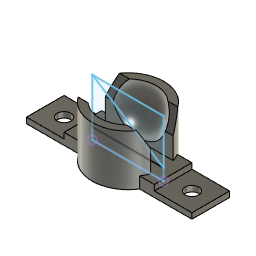
robot (Autodesk Fusion 360 archive; units mm, degrees)
design "Back Caster"
Autodesk Fusion 360 part; units mm, degrees
sketch "Sketch1" plane through (0, 0, 0) normal (0, 0, 1) x (1, 0, 0)
  circle A0 centre (0, 0) radius 9.5
  line L0 (12, 5) -> (-12, 5)
  line L1 (-12, 5) -> (-12, -5)
  line L2 (-12, -5) -> (12, -5)
  line L3 (12, -5) -> (12, 5)
  line L4 (-12, -5) -> (-22, -5)
  line L5 (-22, -5) -> (-22, 5)
  line L6 (-22, 5) -> (-12, 5)
  line L7 (-12, 5) -> (-12, -5)
  line L8 (12, -5) -> (22, -5)
  line L9 (22, -5) -> (22, 5)
  line L10 (22, 5) -> (12, 5)
  line L11 (12, 5) -> (12, -5)
  circle A1 centre (17, 0) radius 1.825
  circle A2 centre (-17, 0) radius 1.825
  dimension "d1" = 19
  dimension "d2" = 5
  dimension "d3" = 5
  dimension "d4" = 12
  dimension "d19" = 24
  dimension "d20" = 3.65
  dimension "d21" = 3.65
  constraint coincident A0.centre origin
  constraint horizontal L0
  constraint vertical L1
  constraint horizontal L2
  constraint vertical L3
  constraint horizontal L4
  constraint vertical L5
  constraint horizontal L6
  constraint vertical L7
  constraint horizontal L8
  constraint vertical L9
  constraint horizontal L10
  constraint vertical L11
  measures "d1" diameter of A0
  measures "d2" distance of A0.centre L0
  measures "d3" distance of A0.centre L2
  measures "d4" distance of A0.centre L3
  measures "d19" distance of L1 L3
  measures "d20" diameter of A1
  measures "d21" diameter of A2
extrude "Extrude1" add sketch "Sketch1" along normal blind 3 contours A0 L0 L2 L3 L11 | A0 L0 L1 L2 L7 makes body 1 at (-9.0078, 3.0183, 2) makes body 2 at (8.3, 4.6217, 2)
extrude "Extrude2" add sketch "Sketch1" along normal blind 13.5 contours A0 L0 L2 | A0 L0 | A0 L2 bodies 1 2
sketch "Sketch2" plane through (0, 0, 0) normal (0, 1, 0) x (1, 0, 0)
  line L0 (-9.5, -15) -> (9.5, -15)
  line L1 (9.5, -15) -> (9.5, 0)
  line L2 (9.5, 0) -> (-9.5, 0)
  line L3 (-9.5, 0) -> (-9.5, -15)
  line L4 (9.5, 0) -> (-9.5, 0)
  line L5 (-9.5, 0) -> (-9.5, -3)
  line L6 (-9.5, -3) -> (9.5, -3)
  line L7 (9.5, -3) -> (9.5, 0)
  line L8 (-9.5, -15) -> (9.5, -3)
  line L9 (-9.5, 0) -> (9.5, 0)
  dimension "d10" = 3
  constraint horizontal L0
  constraint vertical L1
  constraint horizontal L2
  constraint vertical L3
  constraint horizontal L4
  constraint vertical L5
  constraint horizontal L6
  constraint vertical L7
  constraint coincident L3 L5.end
  measures "d10" distance of L6 L9
sphere "SpherePrimitive2" cut diameter 15.8 placed x (1, 0, 0) y (0, 0, -1) z (0, 1, 0) at (0, 0, 11) bodies 1
sketch "Sketch7" plane through (0, 0, 0) normal (1, 0, 0) x (0, 1, 0)
  line L0 (0, 3) -> (-3, 3)
  line L1 (-3, 3) -> (-3, 13.5)
  line L2 (-3, 13.5) -> (0, 13.5)
  line L3 (0, 13.5) -> (0, 3)
  line L4 (-5, 0) -> (-5, 3)
  line L5 (0, 15) -> (0, 0)
  line L6 (0, 3) -> (3, 3)
  line L7 (3, 3) -> (3, 13.5)
  line L8 (0, 13.5) -> (0, 3)
  line L9 (3, 13.5) -> (0, 13.5)
  line L10 (0, 13.5) -> (-5.5, 13.5)
  line L11 (-5.5, 13.5) -> (0, 3)
  line L12 (5.5, 13.5) -> (0, 3)
  line L13 (0, 13.5) -> (5.5, 13.5)
  dimension "d12" = 3
  dimension "d13" = 2
  dimension "d14" = 10.5
  constraint horizontal L0
  constraint vertical L1
  constraint horizontal L2
  constraint vertical L3
  constraint symmetric L0.start L5 L3.end
  constraint symmetric L0.end L5 L6.end
  constraint symmetric L1.end L5 L7.end
  constraint symmetric L2.end L5 L3.start
  constraint perpendicular L1 L10
  constraint symmetric L5 L0.start L3.end
  constraint symmetric L5 L10.end L12.start
  measures "d12" distance of L0.start L0.end
  measures "d13" distance of L1 L4
  measures "d14" distance of L0 L2
extrude "Extrude3" cut sketch "Sketch7" along normal blind 17 bodies 1
extrude "Extrude4" cut sketch "Sketch7" against normal blind 11 bodies 1
extrude "Extrude5" add sketch "Sketch1" along normal blind 1.5 contours L3 L8 L9 L10 L11 | L1 L4 L5 L6 L7 bodies 1
equation "d1 = 15 mm + 4 mm"

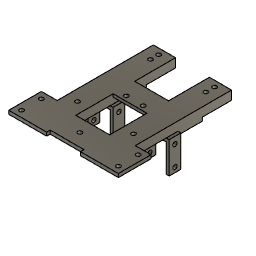
design "Dual Motor Mount"
Autodesk Fusion 360 part; units mm, degrees
sketch "Base" plane through (0, 0, 0) normal (0, 0, 1) x (1, 0, 0)
  line L0 (0, 0) -> (19, 0)
  line L1 (19, 0) -> (19, 31)
  line L2 (19, 31) -> (0, 31)
  line L3 (0, 31) -> (0, 0)
  line L4 (19, 0) -> (21.5, 0)
  line L5 (21.5, 0) -> (21.5, 10)
  line L6 (21.5, 10) -> (19, 10)
  line L7 (19, 10) -> (19, 0)
  line L8 (0, 0) -> (-2.5, 0)
  line L9 (-2.5, 0) -> (-2.5, 10)
  line L10 (-2.5, 10) -> (0, 10)
  line L11 (0, 10) -> (0, 0)
  line L12 (0, 2.5) -> (19, 2.5)
  line L13 (0, 12.6795) -> (0, 2.5)
  line L14 (0, 21) -> (19, 21)
  dimension "d1" = 19
  dimension "d2" = 31
  dimension "d3" = 2.5
  dimension "d4" = 10
  dimension "d5" = 2.5
  dimension "d6" = 10
  dimension "d8" = 2.5
  dimension "d9" = 10
  constraint horizontal L0
  constraint vertical L1
  constraint horizontal L2
  constraint vertical L3
  constraint coincident L0.start L3.end
  constraint horizontal L4
  constraint vertical L5
  constraint horizontal L6
  constraint vertical L7
  constraint horizontal L8
  constraint vertical L9
  constraint horizontal L10
  constraint vertical L11
  constraint coincident L11 L12.start
  constraint coincident L1 L12.end
  constraint vertical L13
  constraint coincident L3 L14.start
  constraint coincident L1 L14.end
  constraint perpendicular L1 L14
  measures "d1" distance of L0.start L0.end
  measures "d2" distance of L0.start L2.end
  measures "d3" distance of L0.end L4.end
  measures "d4" distance of L0.end L6.end
  measures "d5" distance of L0.start L8.end
  measures "d6" distance of L0.start L10.end
  measures "d8" distance of L0 L12
  measures "d9" distance of L2 L14
extrude "Extrude1" add sketch "Base" along normal blind 3 makes body 1
extrude "Extrude2" add sketch "Base" along normal blind 8 separate body contours L1 L3 L7 L11 L12 L13 L14 makes body 2
extrude "Extrude3" add sketch "Base" against normal blind 24 contours L3 L8 L9 L10 L11 L13 | L1 L4 L5 L6 L7 bodies 1 2
sketch "Sensor mount" plane through (0, 0, 8) normal (0, 0, 1) x (-1, 0, 0)
  line L0 (0, -21) -> (0, -2.5)
  line L1 (0, -2.5) -> (-19, -2.5)
  line L2 (-19, -2.5) -> (-19, -21)
  line L3 (-19, -21) -> (0, -21)
  line L4 (-19, -21) -> (-33.5, -21)
  line L5 (-33.5, -21) -> (-33.5, -2.5)
  line L6 (-33.5, -2.5) -> (-19, -2.5)
  line L7 (-19, -2.5) -> (-19, -21)
  line L8 (-33.5, -2.5) -> (-33.5, -21)
  line L9 (-19, -6.5) -> (-33.5, -6.5)
  circle A0 centre (-26.25, -6.5) radius 1.825
  dimension "d16" = 14.5
  dimension "d17" = 18.5
  dimension "d19" = 4
  dimension "d20" = 3.65
  constraint horizontal L4
  constraint vertical L5
  constraint horizontal L6
  constraint vertical L7
  constraint coincident L2.end L3.start
  constraint vertical L8
  constraint coincident L7 L9.start
  constraint coincident L8 L9.end
  constraint perpendicular L8 L9
  constraint midpoint L9 A0.centre
  measures "d16" distance of L2.end L4.end
  measures "d17" distance of L2.end L1.end
  measures "d19" distance of L6 L9
  measures "d20" diameter of A0
extrude "Extrude4" add sketch "Sensor mount" along normal blind 2.6 contours L0 L1 L2 L3 L7 | L2 L4 L5 L7 L8 L9 A0 | L2 L5 L6 L7 L8 L9 A0 bodies 1
sketch "Motor Holes" plane through (21.5, 0, 0) normal (1, 0, 0) x (0, 1, 0)
  line L0 (10, -24) -> (10, 3)
  line L1 (10, 3) -> (0, 3)
  line L2 (0, 3) -> (0, -24)
  line L3 (0, -24) -> (10, -24)
  line L4 (0, 0) -> (10, 0)
  circle A0 centre (5, -2.825) radius 1.825
  line L5 (5, -4.65) -> (5, -18)
  circle A1 centre (5, -19.825) radius 1.825
  line L6 (0, -2.825) -> (3.175, -2.825)
  line L7 (6.825, -2.825) -> (10, -2.825)
  dimension "d25" = 2.825
  dimension "d26" = 3.65
  dimension "d27" = 17
  dimension "d28" = 3.65
  constraint coincident L4.start origin
  constraint coincident L0 L4.end
  constraint perpendicular L0 L4
  constraint coincident L2 L6.start
  constraint coincident L0 L7.end
  constraint perpendicular L0 L6
  constraint perpendicular L5 L6
  constraint coincident A0 L6.end
  constraint collinear L6 L7
  constraint coincident A0.centre L6
  constraint coincident A0 L7.start
  constraint coincident A0 L5.start
  constraint coincident A1 L5.end
  measures "d25" distance of L4 L6
  measures "d26" diameter of A0
  measures "d27" distance of A0.centre A1.centre
  measures "d28" diameter of A1
extrude "Extrude6" cut sketch "Motor Holes" against normal blind 30 contours A0 | A1 bodies 1
sketch "Version" plane through (0, 0, 10.6) normal (0, 0, 1) x (-1, 0, 0)
  circle A0 centre (-26.25, -6.5) radius 1.825
  line L0 (-33.5, -21) -> (0, -21)
  line L1 (0, -21) -> (0, -2.5)
  line L2 (0, -2.5) -> (-33.5, -2.5)
  line L3 (-3, -14) -> (-16, -14) construction
  line L4 (-16, -14) -> (-16, -19) construction
  line L5 (-16, -19) -> (-3, -19) construction
  line L6 (-3, -19) -> (-3, -14) construction
  line L7 (-33.5, -2.5) -> (-33.5, -21)
  dimension "d31" = 8
mirror "Mirror1" about plane through (0, 0, 0) normal (1, 0, 0) of bodies 1 makes body 3
move_body "Move1" bodies 3 to x (1, 0, 0) y (0, 1, 0) z (0, 0, 1) at (67, 0, 0)
combine "Combine1" operation add target body 3 tool bodies 1
sketch "Sketch5" plane through (0, 2.5, 0) normal (0, -1, 0) x (1, 0, 0)
  line L0 (48, 3) -> (67, 3)
  line L1 (67, 3) -> (67, 10.6)
  line L2 (67, 10.6) -> (0, 10.6)
  line L3 (0, 10.6) -> (0, 3)
  line L4 (0, 3) -> (19, 3)
  line L5 (19, 3) -> (19, 8)
  line L6 (19, 8) -> (48, 8)
  line L7 (48, 8) -> (48, 3)
  line L8 (0, 10.6) -> (19, 10.6)
  line L9 (19, 10.6) -> (19, 3)
  line L10 (19, 3) -> (0, 3)
  line L11 (0, 3) -> (0, 10.6)
  line L12 (67, 3) -> (48, 3)
  line L13 (48, 3) -> (48, 10.6)
  line L14 (48, 10.6) -> (67, 10.6)
  line L15 (67, 10.6) -> (67, 3)
  constraint horizontal L8
  constraint vertical L9
  constraint horizontal L10
  constraint vertical L11
  constraint coincident L4.end L5.start
  constraint coincident L2.end L3.start
  constraint horizontal L12
  constraint vertical L13
  constraint horizontal L14
  constraint vertical L15
  constraint coincident L2 L13.end
  constraint coincident L0.end L1.start
extrude "Extrude8" add sketch "Sketch5" along normal blind 32 contours L0 L1 L2 L7 L12 L13 L14 L15 | L2 L3 L4 L5 L8 L9 L10 L11 bodies 3
sketch "Sketch6" plane through (0, 0, 10.6) normal (0, 0, 1) x (-1, 0, 0)
  circle A0 centre (-26.25, -6.5) radius 1.825
  circle A1 centre (-40.75, -6.5) radius 1.825
  line L0 (-67, -21) -> (0, -21)
  line L1 (0, -21) -> (0, 29.5)
  line L2 (0, 29.5) -> (-19, 29.5)
  line L3 (-19, 29.5) -> (-19, -2.5)
  line L4 (-19, -2.5) -> (-48, -2.5)
  line L5 (-48, -2.5) -> (-48, 29.5)
  line L6 (-48, 29.5) -> (-67, 29.5)
  line L7 (-67, 29.5) -> (-67, -21)
  line L8 (-67, 29.5) -> (-77.5, 29.5)
  line L9 (-77.5, 29.5) -> (-77.5, 51.5)
  line L10 (-77.5, 51.5) -> (-67, 51.5)
  line L11 (-67, 51.5) -> (-67, 29.5)
  line L12 (-77.5, 51.5) -> (10.5, 51.5)
  line L13 (10.5, 51.5) -> (10.5, 29.5)
  line L14 (10.5, 29.5) -> (-77.5, 29.5)
  line L15 (-77.5, 29.5) -> (-77.5, 51.5)
  line L16 (10.5, 29.5) -> (8, 29.5)
  line L17 (8, 29.5) -> (8, 32)
  line L18 (8, 32) -> (10.5, 32)
  line L19 (10.5, 32) -> (10.5, 29.5)
  line L20 (10.5, 51.5) -> (8, 51.5)
  line L21 (8, 51.5) -> (8, 49)
  line L22 (8, 49) -> (10.5, 49)
  line L23 (10.5, 49) -> (10.5, 51.5)
  line L24 (-77.5, 51.5) -> (-75, 51.5)
  line L25 (-75, 51.5) -> (-75, 49)
  line L26 (-75, 49) -> (-77.5, 49)
  line L27 (-77.5, 49) -> (-77.5, 51.5)
  line L28 (-77.5, 29.5) -> (-75, 29.5)
  line L29 (-75, 29.5) -> (-75, 32)
  line L30 (-75, 32) -> (-77.5, 32)
  line L31 (-77.5, 32) -> (-77.5, 29.5)
  circle A2 centre (8, 32) radius 1.8
  circle A3 centre (8, 49) radius 1.8
  circle A4 centre (-75, 49) radius 1.8
  circle A5 centre (-75, 32) radius 1.8
  line L32 (10.5, 29.5) -> (-77.5, 51.5)
  circle A6 centre (-33.5, 40.5) radius 1.8
  dimension "d38" = 10.5
  dimension "d39" = 22
  dimension "d40" = 88
  dimension "d41" = 22
  dimension "d42" = 3.6
  dimension "d43" = 3.6
  dimension "d44" = 3.6
  dimension "d45" = 3.6
  dimension "d46" = 3.6
  constraint horizontal L8
  constraint vertical L9
  constraint horizontal L10
  constraint vertical L11
  constraint coincident L6.end L7.start
  constraint horizontal L12
  constraint vertical L13
  constraint horizontal L14
  constraint vertical L15
  constraint horizontal L16
  constraint vertical L17
  constraint horizontal L18
  constraint vertical L19
  constraint horizontal L20
  constraint vertical L21
  constraint horizontal L22
  constraint vertical L23
  constraint horizontal L24
  constraint vertical L25
  constraint horizontal L26
  constraint vertical L27
  constraint horizontal L28
  constraint vertical L29
  constraint horizontal L30
  constraint vertical L31
  constraint coincident L17.end L18.start
  constraint coincident L21.end L22.start
  constraint coincident L25.end L26.start
  constraint coincident L29.end L30.start
  constraint midpoint L32 A6.centre
  measures "d38" distance of L6.end L8.end
  measures "d39" distance of L6.end L10.end
  measures "d40" distance of L9.end L12.end
  measures "d41" distance of L9.end L8.end
  measures "d42" diameter of A2
  measures "d43" diameter of A3
  measures "d44" diameter of A4
  measures "d45" diameter of A5
  measures "d46" diameter of A6
extrude "Extrude9" add sketch "Sketch6" against normal blind 3 contours L2 L6 L11 L14 L17 L32 A6 | L8 L9 L11 L14 L15 L25 L26 L29 L30 A4 A5 L32 | L8 L9 L14 L15 L28 L29 L30 L31 A5 | L10 L11 L12 L25 L32 | L11 L12 L13 L17 L18 L21 L22 A2 A3 L32 A6 | L14 L16 L17 L32 | L10 L12 L24 L25 L32 | L9 L15 L25 L26 L27 A4 L32 | L13 L17 L18 L19 A2 L32 | L12 L13 L20 L21 L22 L23 A3 bodies 3
sketch "Sketch7" plane through (0, 0, 10.6) normal (0, 0, 1) x (-1, 0, 0)
  line L0 (-19, 29.5) -> (-19, -2.5)
  line L1 (-19, -2.5) -> (-48, -2.5)
  line L2 (-48, -2.5) -> (-48, 29.5)
  line L3 (-48, 29.5) -> (-19, 29.5)
  circle A0 centre (8, 32) radius 1.8
  circle A1 centre (-33.5, 40.5) radius 1.8
  circle A2 centre (-75, 49) radius 1.8
  circle A3 centre (-75, 32) radius 1.8
  circle A4 centre (8, 49) radius 1.8
  circle A5 centre (-26.25, -6.5) radius 1.825
  circle A6 centre (-40.75, -6.5) radius 1.825
  line L4 (0, 29.5) -> (10.5, 29.5)
  line L5 (10.5, 29.5) -> (10.5, 51.5)
  line L6 (10.5, 51.5) -> (-77.5, 51.5)
  line L7 (-77.5, 51.5) -> (-77.5, 29.5)
  line L8 (-77.5, 29.5) -> (-67, 29.5)
  line L9 (-67, 29.5) -> (-67, -21)
  line L10 (-67, -21) -> (0, -21)
  line L11 (0, -21) -> (0, 29.5)
  line L12 (0, 29.5) -> (-67, 29.5)
  line L13 (-67, 29.5) -> (-67, 7.5)
  line L14 (-67, 7.5) -> (0, 7.5)
  line L15 (0, 7.5) -> (0, 29.5)
  circle A7 centre (-9.5, 18.5) radius 1.8
  circle A8 centre (-57.5, 18.5) radius 1.8
  circle A9 centre (-9.5, 18.5) radius 5
  circle A10 centre (-57.5, 18.5) radius 5
  line L16 (0, 29.5) -> (-19, 7.5)
  line L17 (-67, 29.5) -> (-48, 7.5)
  line L18 (0, 29.5) -> (0, 51.5)
  line L19 (-67, 29.5) -> (-67, 51.5)
  line L20 (0, 26.5) -> (13.5, 26.5)
  line L21 (13.5, 26.5) -> (13.5, 54.5)
  line L22 (13.5, 54.5) -> (0, 54.5)
  line L23 (0, 54.5) -> (0, 26.5)
  line L24 (10.5, 29.5) -> (-77.5, 29.5)
  line L25 (10.5, 51.5) -> (10.5, 29.5)
  line L26 (-77.5, 51.5) -> (10.5, 51.5)
  line L27 (-67, 26.5) -> (-80.5, 26.5)
  line L28 (-80.5, 26.5) -> (-80.5, 54.5)
  line L29 (-80.5, 54.5) -> (-67, 54.5)
  line L30 (-67, 54.5) -> (-67, 26.5)
  line L31 (-67, 29.5) -> (-77.5, 29.5)
  line L32 (-77.5, 29.5) -> (-77.5, 51.5)
  line L33 (0, 54.5) -> (-19, 54.5)
  line L34 (-19, 54.5) -> (-19, 51.5)
  line L35 (-19, 51.5) -> (0, 51.5)
  line L36 (0, 51.5) -> (0, 54.5)
  line L37 (-67, 54.5) -> (-48, 54.5)
  line L38 (-48, 54.5) -> (-48, 51.5)
  line L39 (-48, 51.5) -> (-67, 51.5)
  line L40 (-67, 51.5) -> (-67, 54.5)
  line L41 (-48, -2.5) -> (-48, 29.5)
  dimension "d49" = 22
  dimension "d50" = 3.6
  dimension "d51" = 3.6
  dimension "d52" = 10
  dimension "d53" = 10
  dimension "d80" = 3
  dimension "d81" = 3
  dimension "d82" = 3
  dimension "d83" = 3
  dimension "d84" = 3
  dimension "d85" = 3
  constraint horizontal L12
  constraint vertical L13
  constraint horizontal L14
  constraint vertical L15
  constraint coincident L4.start L11.end
  constraint concentric A7 A9
  constraint concentric A8 A10
  constraint coincident L0 L16.end
  constraint coincident L14 L16.end
  constraint coincident L14 L17.end
  constraint coincident L2 L17.end
  constraint midpoint A7.centre L16
  constraint midpoint A8.centre L17
  constraint coincident L6 L18.end
  constraint perpendicular L6 L18
  constraint coincident L6 L19.end
  constraint perpendicular L6 L19
  constraint horizontal L20
  constraint vertical L21
  constraint horizontal L22
  constraint vertical L23
  constraint coincident L11 L20.start
  constraint horizontal L27
  constraint vertical L28
  constraint horizontal L29
  constraint vertical L30
  constraint coincident L13 L27.start
  constraint coincident L9 L27.start
  constraint horizontal L33
  constraint vertical L34
  constraint horizontal L35
  constraint vertical L36
  constraint coincident L6 L34.end
  constraint horizontal L37
  constraint vertical L38
  constraint horizontal L39
  constraint vertical L40
  constraint coincident L6 L38.end
  constraint collinear L0 L34
  constraint collinear L38 L41
  measures "d49" distance of L4.start L14.end
  measures "d50" diameter of A7
  measures "d51" diameter of A8
  measures "d52" diameter of A9
  measures "d53" diameter of A10
  measures "d80" distance of L20 L24
  measures "d81" distance of L21 L25
  measures "d82" distance of L22 L26
  measures "d83" distance of L27 L31
  measures "d84" distance of L26 L29
  measures "d85" distance of L28 L32
extrude "Extrude10" cut sketch "Sketch7" against normal blind 8 contours A7 A9 L16 | A7 A9 L16 | A8 A10 L17 | A8 A10 L17 | A7 L16 | A7 L16 | A8 L17 | A8 L17 bodies 3
extrude "Extrude11" add sketch "Sketch7" against normal blind 2.5 contours A7 A9 L16 | A7 A9 L16 | A8 A10 L17 | A8 A10 L17 bodies 3
sketch "Sketch8" plane through (0, 21, 0) normal (0, 1, 0) x (-1, 0, 0)
  line L0 (-67, 3) -> (-48, 3)
  line L1 (-48, 3) -> (-48, 8)
  line L2 (-48, 8) -> (-19, 8)
  line L3 (-19, 8) -> (-19, 3)
  line L4 (-19, 3) -> (0, 3)
  line L5 (0, 3) -> (0, 10.6)
  line L6 (0, 10.6) -> (-67, 10.6)
  line L7 (-67, 10.6) -> (-67, 3)
  line L8 (-67, 10.6) -> (-48, 10.6)
  line L9 (-48, 10.6) -> (-48, 3)
  line L10 (-48, 3) -> (-67, 3)
  line L11 (-67, 3) -> (-67, 10.6)
  line L12 (0, 10.6) -> (-19, 10.6)
  line L13 (-19, 10.6) -> (-19, 3)
  line L14 (-19, 3) -> (0, 3)
  line L15 (0, 3) -> (0, 10.6)
  constraint horizontal L8
  constraint vertical L9
  constraint horizontal L10
  constraint vertical L11
  constraint coincident L0.end L1.start
  constraint coincident L6.end L7.start
  constraint horizontal L12
  constraint vertical L13
  constraint horizontal L14
  constraint vertical L15
  constraint coincident L3.end L4.start
  constraint coincident L5.end L6.start
extrude "Extrude12" add sketch "Sketch8" along normal blind 35 contours L0 L1 L6 L7 L8 L9 L10 L11 | L3 L4 L5 L6 L12 L13 L14 L15 bodies 3
sketch "Sketch9" plane through (0, 0, 3) normal (0, 0, -1) x (1, 0, 0)
  line L0 (67, -31) -> (48, -31)
  line L1 (48, -31) -> (48, -56)
  line L2 (48, -56) -> (67, -56)
  line L3 (67, -56) -> (67, -31)
  line L4 (48, -56) -> (54, -56)
  line L5 (54, -56) -> (54, -31)
  line L6 (54, -31) -> (48, -31)
  line L7 (48, -31) -> (48, -56)
  line L8 (67, -56) -> (61, -56)
  line L9 (61, -56) -> (61, -31)
  line L10 (61, -31) -> (67, -31)
  line L11 (67, -31) -> (67, -56)
  line L12 (54, -56) -> (61, -56)
  line L13 (61, -56) -> (61, -31)
  line L14 (61, -31) -> (54, -31)
  line L15 (54, -31) -> (54, -56)
  line L16 (0.0441, -56) -> (6.0441, -56)
  line L17 (6.0441, -56) -> (6.0441, -31)
  line L18 (6.0441, -31) -> (0.0441, -31)
  line L19 (0.0441, -31) -> (0.0441, -56)
  line L20 (19, -56) -> (13, -56)
  line L21 (13, -56) -> (13, -31)
  line L22 (13, -31) -> (19, -31)
  line L23 (19, -31) -> (19, -56)
  line L24 (6.0441, -56) -> (13.0441, -56)
  line L25 (13.0441, -56) -> (13.0441, -31)
  line L26 (13.0441, -31) -> (6.0441, -31)
  line L27 (6.0441, -31) -> (6.0441, -56)
  line L28 (19, -56) -> (13, -56)
  line L29 (13, -56) -> (13, -31)
  line L30 (13, -31) -> (19, -31)
  line L31 (19, -31) -> (19, -56)
  line L32 (9.5441, -56) -> (9.5441, -51)
  circle A0 centre (9.5441, -51) radius 1.8
  line L33 (9.5441, -51) -> (9.5441, -44)
  circle A1 centre (9.5441, -44) radius 1.8
  line L34 (57.5, -56) -> (57.5, -51)
  circle A2 centre (57.5, -51) radius 1.8
  line L35 (57.5, -51) -> (57.5, -43.5)
  circle A3 centre (57.5, -43.5) radius 1.8
  dimension "d60" = 6
  dimension "d61" = 6
  dimension "d62" = 6
  dimension "d64" = 6
  dimension "d65" = 5
  dimension "d66" = 3.6
  dimension "d67" = 3.6
  dimension "d68" = 3.6
  dimension "d69" = 3.6
  constraint horizontal L4
  constraint vertical L5
  constraint horizontal L6
  constraint vertical L7
  constraint coincident L1.end L2.start
  constraint horizontal L8
  constraint vertical L9
  constraint horizontal L10
  constraint vertical L11
  constraint coincident L2.end L3.start
  constraint horizontal L12
  constraint vertical L13
  constraint horizontal L14
  constraint vertical L15
  constraint horizontal L16
  constraint vertical L17
  constraint horizontal L18
  constraint vertical L19
  constraint horizontal L20
  constraint vertical L21
  constraint horizontal L22
  constraint vertical L23
  constraint horizontal L24
  constraint vertical L25
  constraint horizontal L26
  constraint vertical L27
  constraint horizontal L28
  constraint vertical L29
  constraint horizontal L30
  constraint vertical L31
  constraint midpoint L24 L32.start
  constraint perpendicular L24 L32
  constraint coincident L32.end A0.centre
  constraint perpendicular L24 L33
  constraint coincident L33.end A1.centre
  constraint midpoint L2 L34.start
  constraint perpendicular L2 L34
  constraint coincident L34.end A2.centre
  constraint parallel L34 L35
  constraint coincident L35.end A3.centre
  measures "d60" distance of L1.end L4.end
  measures "d61" distance of L2.end L8.end
  measures "d62" distance of L16.start L16.end
  measures "d64" distance of L21 L31
  measures "d65" distance of L32.start L32.end
  measures "d66" diameter of A0
  measures "d67" diameter of A1
  measures "d68" diameter of A2
  measures "d69" diameter of A3
extrude "Extrude13" cut sketch "Sketch9" against normal blind 4.6 contours L0 L2 L5 L9 L12 L13 L14 L15 | L17 L21 L24 L26 L27 L29 | L32 A0 L33 | L32 A0 L33 | A1 | L34 A2 L35 | L34 A2 L35 | A3 bodies 3
extrude "Extrude14" cut sketch "Sketch9" against normal blind 9 contours L32 A0 L33 | L32 A0 L33 | A1 | L34 A2 L35 | L34 A2 L35 | A3 bodies 3
sketch "Sketch10" plane through (67, 0, 0) normal (1, 0, 0) x (0, 1, 0)
  line L0 (31, 3) -> (56, 3)
  line L1 (56, 3) -> (56, 10.6)
  line L2 (56, 10.6) -> (-29.5, 10.6)
  line L3 (-29.5, 10.6) -> (-29.5, 7.6)
  line L4 (-29.5, 7.6) -> (-29.5, 3)
  line L5 (-29.5, 3) -> (0, 3)
  line L6 (0, 3) -> (10, 3)
  line L7 (10, 3) -> (10, 0)
  line L8 (10, 0) -> (31, 0)
  line L9 (31, 0) -> (31, 3)
  line L10 (-29.5, 3) -> (-29.5, 7.6)
  line L11 (-29.5, 3) -> (-51.5, 3)
  line L12 (-51.5, 3) -> (-51.5, 7.6)
  line L13 (-51.5, 7.6) -> (-29.5, 7.6)
  line L14 (-29.5, 7.6) -> (-29.5, 3)
  line L15 (-51.5, 7.6) -> (-29.5, 3)
  dimension "d74" = 22
  constraint coincident L4.end L5.start
  constraint coincident L3.end L4.start
  constraint horizontal L11
  constraint vertical L12
  constraint horizontal L13
  constraint vertical L14
  measures "d74" distance of L4.end L11.end
extrude "Extrude15" add sketch "Sketch10" against normal blind 19 contours L4 L10 L13 L14 L15 bodies 3
sketch "Sketch11" plane through (0, 0, 0) normal (-1, 0, 0) x (0, -1, 0)
  line L0 (-31, 3) -> (-31, 0)
  line L1 (-31, 0) -> (-10, 0)
  line L2 (-10, 0) -> (-10, 3)
  line L3 (-10, 3) -> (0, 3)
  line L4 (0, 3) -> (29.5, 3)
  line L5 (29.5, 3) -> (29.5, 7.6)
  line L6 (29.5, 7.6) -> (29.5, 10.6)
  line L7 (29.5, 10.6) -> (-56, 10.6)
  line L8 (-56, 10.6) -> (-56, 3)
  line L9 (-56, 3) -> (-31, 3)
  line L10 (29.5, 3) -> (51.5, 3)
  line L11 (51.5, 3) -> (51.5, 7.6)
  line L12 (51.5, 7.6) -> (29.5, 7.6)
  line L13 (29.5, 7.6) -> (29.5, 3)
  line L14 (29.5, 3) -> (51.5, 7.6)
  dimension "d77" = 22
  constraint horizontal L10
  constraint vertical L11
  constraint horizontal L12
  constraint vertical L13
  constraint coincident L4.end L5.start
  measures "d77" distance of L4.end L10.end
extrude "Extrude16" add sketch "Sketch11" against normal blind 19 contours L5 L12 L13 L14 bodies 3
extrude "Extrude17" add sketch "Sketch7" against normal blind 3 contours L4 L5 L6 L11 L15 L20 L21 L22 L23 L24 L25 L26 L36 | L6 L7 L8 L9 L13 L24 L26 L27 L28 L29 L30 L31 L32 L40 | L6 L23 L26 L33 L34 L35 L36 | L6 L26 L30 L37 L38 L39 L40 bodies 3
equation "d38 = ( ( 88 - 67 ) / 2 ) * 1 mm"
equation "d49 = 16 mm + 6 mm"
equation "d70 = 3 mm - 7.6 mm"

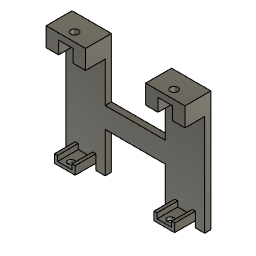
design "IR Front Mount"
Autodesk Fusion 360 part; units mm, degrees
sketch "Top Screw Holes" plane through (0, 0, 0) normal (0, 0, 1) x (1, 0, 0)
  line L0 (0, 0) -> (19, 0)
  line L1 (19, 0) -> (19, 9.5)
  line L2 (19, 9.5) -> (0, 9.5)
  line L3 (0, 9.5) -> (0, 0)
  line L4 (33.5, 0) -> (33.5, 8.5)
  circle A0 centre (9.5, 4.25) radius 1.825
  line L5 (0, 9.5) -> (19, 9.5)
  line L6 (19, 9.5) -> (19, 12.5)
  line L7 (19, 12.5) -> (0, 12.5)
  line L8 (0, 12.5) -> (0, 9.5)
  line L9 (0, 0) -> (6, 0)
  line L10 (6, 0) -> (6, 9.5)
  line L11 (6, 9.5) -> (1.0556, 9.5)
  line L12 (0, 8.5) -> (0, 0)
  line L13 (19, 0) -> (13, 0)
  line L14 (13, 0) -> (13, 9.5)
  line L15 (13, 9.5) -> (19, 9.5)
  line L16 (19, 9.5) -> (19, 0)
  line L17 (1.0556, 9.5) -> (19, 9.5)
  line L18 (19, 9.5) -> (19, 8.5)
  line L19 (0, 9.5) -> (19, 9.5)
  line L20 (19, 9.5) -> (19, 8.5)
  line L21 (19, 8.5) -> (0, 8.5)
  line L22 (0, 8.5) -> (0, 9.5)
  line L23 (19, 0) -> (0, 8.5)
  line L24 (48, 0) -> (48, 9.5)
  line L25 (65.9444, 9.5) -> (48, 9.5)
  line L26 (61, 0) -> (61, 9.5)
  line L27 (48, 9.5) -> (48, 8.5)
  line L28 (48, 8.5) -> (67, 8.5)
  line L29 (67, 0) -> (48, 0)
  line L30 (48, 12.5) -> (67, 12.5)
  line L31 (67, 9.5) -> (48, 9.5)
  line L32 (61, 9.5) -> (65.9444, 9.5)
  line L33 (67, 8.5) -> (67, 0)
  line L34 (67, 8.5) -> (67, 9.5)
  line L35 (67, 0) -> (61, 0)
  line L36 (48, 9.5) -> (48, 8.5)
  line L37 (67, 12.5) -> (67, 9.5)
  line L38 (67, 9.5) -> (48, 9.5)
  line L39 (48, 0) -> (67, 8.5)
  line L40 (48, 9.5) -> (48, 0)
  line L41 (54, 9.5) -> (48, 9.5)
  line L42 (67, 9.5) -> (67, 0)
  line L43 (48, 9.5) -> (48, 12.5)
  line L44 (48, 0) -> (54, 0)
  circle A1 centre (57.5, 4.25) radius 1.825
  line L45 (48, 9.5) -> (67, 9.5)
  line L46 (54, 0) -> (54, 9.5)
  point P0 (67, 0)
  dimension "d1" = 19
  dimension "d2" = 9.5
  dimension "d3" = 14.5
  dimension "d5" = 3.65
  dimension "d6" = 3
  dimension "d7" = 6
  dimension "d8" = 6
  dimension "d37" = 1
  constraint horizontal L0
  constraint vertical L1
  constraint horizontal L2
  constraint vertical L3
  constraint coincident L0.start L3.end
  constraint perpendicular L2 L4
  constraint horizontal L5
  constraint vertical L6
  constraint horizontal L7
  constraint vertical L8
  constraint horizontal L9
  constraint vertical L10
  constraint horizontal L11
  constraint vertical L12
  constraint horizontal L13
  constraint vertical L14
  constraint horizontal L15
  constraint vertical L16
  constraint equal L3 L10
  constraint equal L1 L14
  constraint horizontal L17
  constraint vertical L18
  constraint horizontal L19
  constraint vertical L20
  constraint horizontal L21
  constraint vertical L22
  constraint midpoint A0.centre L23
  constraint symmetric L0.start L4 L29.start
  constraint symmetric L0.start L4 P0
  constraint symmetric L0.end L4 L24.start
  constraint symmetric L1.end L4 L24.end
  constraint symmetric L2.end L4 L31.start
  constraint symmetric L4 A0 A1
  constraint symmetric L4 L1.end L24.end
  constraint symmetric L4 L6.end L30.start
  constraint symmetric L4 L7.end L30.end
  constraint symmetric L4 L0.start P0
  constraint symmetric L4 L9.end L26.start
  constraint symmetric L4 L10.end L26.end
  constraint symmetric L4 L12.start L28.end
  constraint symmetric L4 L13.end L44.end
  constraint symmetric L4 L14.end L41.start
  constraint symmetric L4 L11.end L25.start
  constraint symmetric L4 L18.end L27.end
  measures "d1" distance of L0.start L0.end
  measures "d2" distance of L0.start L2.end
  measures "d3" distance of L1 L4
  measures "d5" diameter of A0
  measures "d6" distance of L2.end L7.end
  measures "d7" distance of L0.start L9.end
  measures "d8" distance of L0.end L13.end
  measures "d37" distance of L2.end L12.start
extrude "Extrude1" add sketch "Top Screw Holes" along normal blind 3 contours L0 L3 L9 L10 L12 L23 | L0 A0 L10 L14 L23 | L2 L3 L5 L10 L11 L17 L19 L21 L22 | L10 L21 L23 | L0 L13 L14 L23 | A0 L10 L14 L21 L23 | L2 L5 L6 L7 L8 L11 L15 L17 L19 | L2 L5 L10 L14 L17 L19 L21 | L1 L14 L16 L21 L23 | L1 L2 L5 L14 L15 L16 L17 L18 L19 L20 L21 | L29 L39 L44 L46 | L24 L28 L39 L40 L46 | L24 L25 L27 L28 L31 L36 L38 L40 L41 L45 L46 | L26 L29 L39 A1 L46 | L26 L28 L39 A1 L46 | L25 L30 L31 L32 L37 L38 L41 L43 L45 | L25 L26 L28 L31 L38 L45 L46 | L26 L29 L33 L35 L39 L42 | L26 L28 L39 | L25 L26 L28 L31 L32 L34 L38 L42 L45 makes body 1 at (2.5854, 5.7626, 0) makes body 2 at (64.4146, 5.7626, 0)
extrude "Extrude2" add sketch "Top Screw Holes" against normal blind 6.2 separate body contours L0 L3 L9 L10 L12 L23 | L2 L3 L5 L10 L11 L17 L19 L21 L22 | L10 L21 L23 | L0 L13 L14 L23 | L1 L14 L16 L21 L23 | L1 L2 L5 L14 L15 L16 L17 L18 L19 L20 L21 | L29 L39 L44 L46 | L24 L28 L39 L40 L46 | L24 L25 L27 L28 L31 L36 L38 L40 L41 L45 L46 | L26 L29 L33 L35 L39 L42 | L26 L28 L39 | L25 L26 L28 L31 L32 L34 L38 L42 L45 makes body 3 at (0, 6.3333, -2.0667) makes body 4 at (48, 3.1667, -2.0667) makes body 5 at (19, 3.1667, -2.0667) makes body 6 at (61, 3.1667, -2.0667)
extrude "Extrude3" add sketch "Top Screw Holes" against normal blind 55 contours L2 L5 L6 L7 L8 L11 L15 L17 L19 | L25 L30 L31 L32 L37 L38 L41 L43 L45 bodies 2 5 4 6 3 1
sketch "H-Cross" plane through (19, 0, 0) normal (1, 0, 0) x (0, 1, 0)
  line L0 (12.5, -55) -> (12.5, 3)
  line L1 (12.5, 3) -> (0, 3)
  line L2 (0, 3) -> (0, -6.2)
  line L3 (0, -6.2) -> (9.5, -6.2)
  line L4 (9.5, -6.2) -> (9.5, -55)
  line L5 (9.5, -55) -> (12.5, -55)
  line L6 (12.5, -25.6) -> (9.5, -25.6)
  line L7 (9.5, -25.6) -> (9.5, -35.6)
  line L8 (9.5, -35.6) -> (12.5, -35.6)
  line L9 (12.5, -35.6) -> (12.5, -25.6)
  dimension "d15" = 10
  constraint horizontal L6
  constraint vertical L7
  constraint horizontal L8
  constraint vertical L9
  constraint coincident L0 L6.start
  constraint midpoint L4 L7
  measures "d15" distance of L6.start L8.end
extrude "Extrude4" add sketch "H-Cross" along normal blind 29 contours L0 L4 L6 L7 L8 L9 bodies 2 5
sketch "Bottom Notches" plane through (0, 0, -55) normal (0, 0, -1) x (1, 0, 0)
  line L0 (67, -9.5) -> (48, -9.5)
  line L1 (48, -12.5) -> (67, -12.5)
  line L2 (4.5, -12.5) -> (14.5, -12.5)
  line L3 (14.5, -12.5) -> (14.5, -8.5)
  line L4 (14.5, -8.5) -> (4.5, -8.5)
  line L5 (4.5, -8.5) -> (4.5, -12.5)
  line L6 (19, -12.5) -> (0, -12.5)
  line L7 (33.5, 0) -> (33.5, -8.5)
  line L8 (62.5, -12.5) -> (52.5, -12.5)
  line L9 (52.5, -8.5) -> (62.5, -8.5)
  line L10 (52.5, -12.5) -> (52.5, -8.5)
  line L11 (62.5, -8.5) -> (62.5, -12.5)
  line L12 (48, -12.5) -> (67, -12.5)
  line L13 (0, -9.5) -> (0, -12.5)
  line L14 (19, -12.5) -> (19, -9.5)
  line L15 (48, -9.5) -> (48, -12.5)
  line L16 (67, -12.5) -> (67, -9.5)
  line L17 (19, -9.5) -> (0, -9.5)
  line L18 (0, -12.5) -> (19, -12.5)
  dimension "d18" = 10
  constraint horizontal L2
  constraint vertical L3
  constraint horizontal L4
  constraint vertical L5
  constraint midpoint L2 L6
  constraint symmetric L2.start L7 L8.start
  constraint symmetric L2.end L7 L8.end
  constraint symmetric L3.end L7 L9.start
  constraint symmetric L4.end L7 L9.end
  constraint symmetric L6.start L7 L1.start
  constraint symmetric L6.end L7 L1.end
  measures "d18" distance of L2.start L2.end
extrude "Extrude5" cut sketch "Bottom Notches" against normal blind 3 contours L0 L1 L8 L10 L11 L12 | L0 L9 L10 L11 | L2 L3 L5 L6 L17 L18 | L3 L4 L5 L17 bodies 2
sketch "Bottom Screw Mount" plane through (0, 9.5, 0) normal (0, -1, 0) x (1, 0, 0)
  line L0 (61, 0) -> (54, 0)
  line L1 (48, -25.6) -> (19, -25.6)
  line L2 (19, -25.6) -> (19, -6.2)
  line L3 (67, -6.2) -> (61, -6.2)
  line L4 (13, -6.2) -> (13, 0)
  line L5 (0, -6.2) -> (0, -55)
  line L6 (62.5, -55) -> (67, -55)
  line L7 (4.5, -55) -> (4.5, -52)
  line L8 (4.5, -52) -> (14.5, -52)
  line L9 (14.5, -52) -> (14.5, -55)
  line L10 (19, -35.6) -> (48, -35.6)
  line L11 (4.5, -52) -> (14.5, -52)
  line L12 (14.5, -52) -> (14.5, -50.5)
  line L13 (14.5, -50.5) -> (4.5, -50.5)
  line L14 (4.5, -50.5) -> (4.5, -52)
  line L15 (4.5, -52) -> (6, -52)
  line L16 (6, -52) -> (6, -48)
  line L17 (6, -48) -> (4.5, -48)
  line L18 (4.5, -48) -> (4.5, -52)
  line L19 (14.5, -52) -> (13, -52)
  line L20 (13, -52) -> (13, -48)
  line L21 (13, -48) -> (14.5, -48)
  line L22 (14.5, -48) -> (14.5, -52)
  line L23 (33.5, -25.6) -> (33.5, -35.6)
  line L24 (61, -52) -> (61, -48)
  line L25 (52.5, -48) -> (52.5, -52)
  line L26 (62.5, -48) -> (62.5, -52)
  line L27 (52.5, -52) -> (54, -52)
  line L28 (52.5, -50.5) -> (62.5, -50.5)
  line L29 (52.5, -52) -> (52.5, -50.5)
  line L30 (62.5, -52) -> (52.5, -52)
  line L31 (54, -52) -> (54, -48)
  line L32 (62.5, -55) -> (62.5, -52)
  line L33 (62.5, -52) -> (61, -52)
  line L34 (61, -48) -> (62.5, -48)
  line L35 (54, -48) -> (52.5, -48)
  line L36 (62.5, -50.5) -> (62.5, -52)
  line L37 (52.5, -52) -> (52.5, -55)
  line L38 (62.5, -52) -> (52.5, -52)
  line L39 (6, 0) -> (6, -6.2)
  line L40 (62.5, -52) -> (62.5, -55)
  line L41 (67, -55) -> (67, -6.2)
  line L42 (61, -6.2) -> (61, 0)
  line L43 (54, 0) -> (54, -6.2)
  line L44 (54, -6.2) -> (48, -6.2)
  line L45 (48, -6.2) -> (48, -25.6)
  line L46 (19, -6.2) -> (13, -6.2)
  line L47 (13, 0) -> (6, 0)
  line L48 (6, -6.2) -> (0, -6.2)
  line L49 (0, -55) -> (4.5, -55)
  line L50 (14.5, -55) -> (19, -55)
  line L51 (19, -55) -> (19, -35.6)
  line L52 (48, -35.6) -> (48, -55)
  line L53 (48, -55) -> (52.5, -55)
  line L54 (52.5, -55) -> (52.5, -52)
  line L55 (52.5, -52) -> (62.5, -52)
  dimension "d21" = 1.5
  dimension "d22" = 1.5
  dimension "d23" = 4
  constraint horizontal L11
  constraint vertical L12
  constraint horizontal L13
  constraint vertical L14
  constraint coincident L7.end L8.start
  constraint horizontal L15
  constraint vertical L16
  constraint horizontal L17
  constraint vertical L18
  constraint horizontal L19
  constraint vertical L20
  constraint horizontal L21
  constraint vertical L22
  constraint midpoint L1 L23.start
  constraint midpoint L10 L23.end
  constraint symmetric L7.start L23 L6.start
  constraint symmetric L7.end L23 L26.end
  constraint symmetric L8.end L23 L25.end
  constraint symmetric L9.end L23 L37.end
  constraint symmetric L12.end L23 L28.start
  constraint symmetric L13.end L23 L28.end
  constraint symmetric L15.end L23 L24.start
  constraint symmetric L16.end L23 L24.end
  constraint symmetric L17.end L23 L26.start
  constraint symmetric L19.end L23 L27.end
  constraint symmetric L20.end L23 L31.end
  constraint symmetric L21.end L23 L25.start
  constraint equal L16 L20
  measures "d21" distance of L7.end L13.end
  measures "d22" distance of L7.end L15.end
  measures "d23" distance of L7.end L17.end
extrude "Extrude6" add sketch "Bottom Screw Mount" along normal blind 10 contours L24 L26 L28 L30 L33 L36 L38 L55 | L24 L26 L28 L34 | L24 L28 L30 L31 L38 L55 | L25 L27 L28 L29 L30 L31 L38 L55 | L25 L28 L31 L35 | L8 L11 L12 L13 L19 L20 L22 | L8 L11 L13 L16 L20 | L13 L20 L21 L22 | L8 L11 L13 L14 L15 L16 L18 | L13 L16 L17 L18 bodies 2
sketch "Bottom Screw Hole" plane through (0, 0, -50.5) normal (0, 0, 1) x (-1, 0, 0)
  line L0 (-13, -9.5) -> (-6, -9.5)
  line L1 (-6, -9.5) -> (-6, 0.5)
  line L2 (-6, 0.5) -> (-13, 0.5)
  line L3 (-13, 0.5) -> (-13, -9.5)
  line L4 (-6, -9.5) -> (-13, -9.5)
  line L5 (-13, -9.5) -> (-13, -5.5)
  line L6 (-13, -5.5) -> (-6, -5.5)
  line L7 (-6, -5.5) -> (-6, -9.5)
  line L8 (-6, -5.5) -> (-13, 0.5)
  circle A0 centre (-9.5, -2.5) radius 1.5825
  line L9 (-13, -9.5) -> (-54, -9.5)
  line L10 (-33.5, -9.5) -> (-33.5, -1)
  line L11 (-54, -9.5) -> (-61, -9.5)
  line L12 (-54, -5.5) -> (-61, -5.5)
  line L13 (-61, 0.5) -> (-54, 0.5)
  circle A1 centre (-57.5, -2.5) radius 1.5825
  line L14 (-54, -9.5) -> (-54, -5.5)
  line L15 (-61, -9.5) -> (-61, 0.5)
  line L16 (-61, -5.5) -> (-61, -9.5)
  line L17 (-54, 0.5) -> (-54, -9.5)
  line L18 (-61, -5.5) -> (-54, 0.5)
  line L19 (-61, -9.5) -> (-54, -9.5)
  point P0 (-67, 0)
  point P1 (-54, -9.5)
  dimension "d30" = 4
  dimension "d31" = 3.165
  constraint horizontal L4
  constraint vertical L5
  constraint horizontal L6
  constraint vertical L7
  constraint coincident L0.end L1.start
  constraint coincident L2.end L3.start
  constraint midpoint L8 A0.centre
  constraint coincident L0.start L3.end
  constraint perpendicular L5 L9
  constraint midpoint L9 L10.start
  constraint perpendicular L9 L10
  constraint symmetric origin L10 P0
  constraint symmetric L0.start L10 L9.end
  constraint symmetric L0.end L10 L11.end
  constraint symmetric L1.end L10 L13.start
  constraint symmetric L2.end L10 L13.end
  constraint symmetric L0.start L10 P1
  constraint symmetric L5.end L10 L12.start
  constraint symmetric L6.end L10 L12.end
  constraint symmetric A0 L10 A1
  measures "d30" distance of L0.end L6.end
  measures "d31" diameter of A0
extrude "Extrude8" cut sketch "Bottom Screw Hole" against normal blind 1.5 contours L8 A0 | L8 A0 | A1 L18 | A1 L18 bodies 2
equation "d3 = ( 29 / 2 ) * 1 mm"
named bodies: "IR Front Mount"
